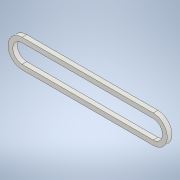
# Autodesk Inventor part: カウンター固定具
Saved by Autodesk Inventor 2020.2 (Build 242310000, 310)
## iProperties
Created: 2020-04-03
Part Number: カウンター固定具
Material: 鋼、非合金鋼
Document SubType Name: Modeling
Designer: aoyama
Density: 7.85 g/cm^3
Appearance: 鋼
Author: aoyama
Autodesk Inventor part; units mm, degrees
ref_plane "YZ Plane" through (0, 0, 0) normal (1, 0, 0) x (0, 1, 0)
ref_plane "XZ Plane" through (0, 0, 0) normal (0, 1, 0) x (-1, 0, 0)
ref_plane "XY Plane" through (0, 0, 0) normal (0, 0, 1) x (1, 0, 0)
sketch "スケッチ1" plane through (0, 0, 0) normal (0, 0, 1) x (1, 0, 0)
  line L0 (0, 0) -> (-28, 0) construction
  line L1 (0, 3) -> (-28, 3)
  line L2 (-28, -3) -> (0, -3)
  arc A0 (0, -3) -> (0, 3) centre (0, 0) ccw
  arc A1 (-28, 3) -> (-28, -3) centre (-28, 0) ccw
  line L3 (-28, 2) -> (0, 2)
  arc A2 (0, -2) -> (0, 2) centre (0, 0) ccw
  line L4 (0, -2) -> (-28, -2)
  arc A3 (-28, 2) -> (-28, -2) centre (-28, 0) ccw
  point P0 (-14, 0)
  dimension "d0" = 6
  dimension "d1" = 28
  dimension "d2" = 1
  constraints: 12 end point, 8 point on circle, 4 centre point, 4 tangent, 2 parallel, 1 midpoint, 3 other
  measures "d0" diameter of A1
  measures "d1" distance of L0.start L0.end
  measures "d2" distance between parallel lines of L1 L3
extrude "押し出し1" add sketch "スケッチ1" along normal blind 1
